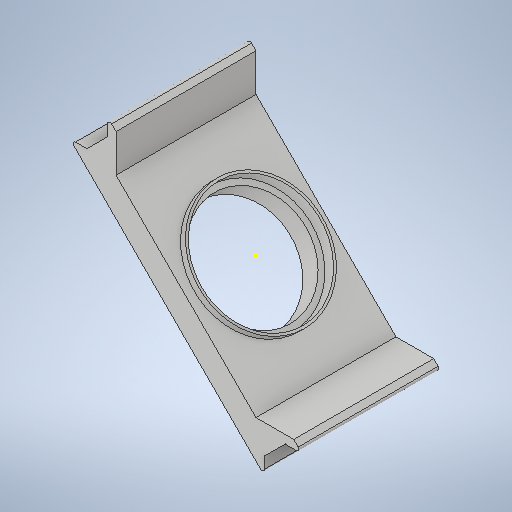
# Autodesk Inventor part: fenguangjing
Saved by Autodesk Inventor 2025.1 (Build 291241000, 241)
## iProperties
Created: 2024-08-22
Part Number: fenguangjing
Material: Generic
Document SubType Name: Sheet Metal
Designer: Administrator
Density: 1 g/cm^3
Sheet Metal Rule: 默认_mm
Appearance: Default
Author: Administrator
Autodesk Inventor part; units mm, degrees
note: some values were not read from the file. Chosen so that the rebuilt part matches the saved one: direction of "孔2".
ref_plane "YZ Plane" through (0, 0, 0) normal (1, 0, 0) x (0, 1, 0)
ref_plane "XZ Plane" through (0, 0, 0) normal (0, 1, 0) x (-1, 0, 0)
ref_plane "XY Plane" through (0, 0, 0) normal (0, 0, 1) x (1, 0, 0)
sketch "草图1" plane through (0, 0, 0) normal (0, 0, 1) x (1, 0, 0)
  line L0 (-16.8, 24.9) -> (-16.8, 21.24)
  line L1 (-16.8, 21.24) -> (-21.2406, 16.7994)
  line L2 (-21.2406, 16.7994) -> (-24.9006, 16.7994)
  line L3 (16.8, -24.9) -> (16.8, -21.24)
  line L4 (16.8, -21.24) -> (21.2406, -16.7994)
  line L5 (21.2406, -16.7994) -> (24.9006, -16.7994)
  line L6 (-24.9006, 16.7994) -> (16.8, -24.9)
  line L7 (0, 0) -> (-0.1347, -0.1347)
  line L8 (22.4746, -22.7439) -> (22.4746, -22.7439)
  line L9 (-15, 15) -> (-15, 23.1001)
  line L10 (15, -15) -> (23.1012, -15)
  line L11 (-15, 23.1001) -> (-16.8, 24.9)
  line L12 (23.1012, -15) -> (24.9006, -16.7994)
  line L13 (-15, 15) -> (15, -15)
  constraints: 28 end point, 2 perpendicular, 2 vertical, 1 horizontal
extrude "拉伸1" add sketch "草图1" along normal blind 15 and the other way blind 15
sketch "草图2" plane through (-15, 15, -15) normal (0.7071068, 0.7071068, 0) x (-0.7071068, 0.7071068, 0)
  point P0 (-21.2132, 15)
  point P1 (-21.2132, 15)
  constraints: 1 coincident
hole "孔1" at (0, 0, 0) direction (-0.7071068, -0.7071068, 0) diameter 23 end through all counterbore diameter 25.4 counterbore depth 1.1
sketch "草图3" plane through (-15, 15, -15) normal (0.7071068, 0.7071068, 0) x (-0.7071068, 0.7071068, 0)
  point P0 (-21.2132, 15)
sketch "草图4" plane through (-15, 15, -15) normal (0.7071068, 0.7071068, 0) x (-0.7071068, 0.7071068, 0)
  point P0 (-21.2132, 15)
sketch "草图5" plane through (-15, 15, -15) normal (0.7071068, 0.7071068, 0) x (-0.7071068, 0.7071068, 0)
  circle A0 centre (-21.2132, 15) radius 12.7
  circle A1 centre (-21.2132, 15) radius 13.2
  dimension "d18" = 0.5
  dimension "d19" = 25.4
  constraints: 4 coincident, 2 centre point
  measures "d18" radial gap between concentric circles of A1 A0
  measures "d19" diameter of A0
extrude "拉伸2" add sketch "草图5" along normal blind 1.5 contours A0 | A1
sketch "草图6" plane through (1.0607, 1.0607, 0) normal (0.7071068, 0.7071068, 0) x (-0.7071068, 0.7071068, 0)
  point P0 (0, 0)
  point P1 (0, 0)
  constraints: 1 coincident
hole "孔2" at (1.0607, 1.0607, 0) direction (-0.7071068, -0.7071068, 0) diameter 25.4 end up to surface
fillet "圆角1" radius 0.5 1 edges at (-16.8, 24.9, 0)
fillet "圆角2" radius 0.5 1 edges at (-24.9006, 16.7994, 0)
fillet "圆角3" radius 0.5 1 edges at (24.9006, -16.7994, 0)
fillet "圆角4" radius 0.5 1 edges at (16.8, -24.9, 0)
sketch "草图7" plane through (-15, 15, -15) normal (0.7071068, 0.7071068, 0) x (-0.7071068, 0.7071068, 0)
  point P0 (-21.2132, 15)
equation "\"d15\" = Thickness"
equation "\"BendRadius\" = Thickness"
equation "\"BendReliefWidth\" = Thickness"
equation "\"BendReliefDepth\" = 0.5 * Thickness"
equation "\"CornerReliefSize\" = 4 * Thickness"
equation "\"MinimumRemnant\" = 2 * Thickness"
equation "\"TransitionRadius\" = BendRadius"
equation "\"JacobiRadiusSize\" = BendRadius"
equation "\"GapSize\" = Thickness"
equation "\"Thickness\" = 0.5"
